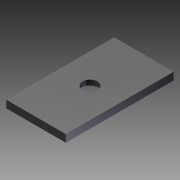
# Autodesk Inventor part: HMEN5-5-dps
Saved by Autodesk Inventor 2015 SP1 (Build 190203100, 203)
## iProperties
Category: Hardware
Company: MISUMI
Created: 2015-02-01
Part Number: HMEN5-5-dps
Catalog Web Link: http://us.misumi-ec.com/vona2/detail/110300479530
Description: HMEN, HMER-door side plate-Latch Magnets for Plate
Vendor: MISUMI
Document SubType Name: Modeling
Designer: psAdmin
Manufacturer: MISUMI
Mass: 0.89831 g
Surface Area: 11.0294 cm^2
Volume: 0.89831 cm^3
Density: 1 g/cm^3
Material: Generic
Appearance: PSOLRGB-192-192-192
Stock Number: HMEN5-5
PSOL_IDENT_0: {\\10.0.0.236\data_v8\23d-libs\misumi\metric\39_accessories_for_al_extrusions\hmen_door_side_plate.p
PSOL_IDENT_1: rj},186 {VTYP=3D},{NB=HMEN5-5-dps},{LINA=HMEN5-5-dps},{NN=HMEN, HMER-door side plate},{DATE=17.11.20
PSOL_IDENT_2: 14 05:31:12},{GEOMDATE=25.05.2009 11:35:00},{VERSION=},{LINEID=10},{LINESUBID=-1},{WBVAR=TS}  {NB=HM
PSOL_IDENT_3: EN5-5-dps},{LINA=HMEN5-5-dps},{KT=DUMMY},{PN=HMEN5-5},{TYPE=HMEN},{TS=HMEN},{NO=5-5}
SUPPLIER: MISUMI
ARTICLENO: HMEN5-5-dps
BOMINFO: HMEN5-5-dps
CREATOR: CADENAS GmbH
Title: HMEN5-5-dps
Author: Misumi
Comments: Latch Magnets for Plate
Autodesk Inventor part; units mm, degrees
sketch "Sketch_1" plane through (0, 0, 0) normal (0, 0, 1) x (1, 0, 0)
  line L0 (-8, 14.5) -> (-8, -14.5)
  line L1 (-8, -14.5) -> (8, -14.5)
  line L2 (8, -14.5) -> (8, 14.5)
  line L3 (8, 14.5) -> (-8, 14.5)
  constraints: 8 end point
extrude "Extrusion1" add sketch "Sketch_1" against normal blind 2
sketch "Sketch_2" plane through (0, 0, 0) normal (1, 0, 0) x (0, 1, 0)
  line L0 (0, -2) -> (0, 0)
  line L1 (0, 0) -> (2, 0)
  line L2 (2, 0) -> (2, -1.2)
  line L3 (2, -1.2) -> (2.8, -2)
  line L4 (2.8, -2) -> (0, -2)
  line L5 (0, -2) -> (0, 0)
  constraints: 12 end point
revolve "Revolution1" cut sketch "Sketch_2" angle 360 about axis through (0, 0, -2) along (0, 0, -1)
ref_plane "to_magnet_XY" through (0, 0, 0) normal (0, 0, 1) x (1, 0, 0)
ref_plane "to_magnet_YZ" through (0, 0, 0) normal (1, 0, 0) x (0, 1, 0)
ref_plane "to_magnet_ZX" through (0, 0, 0) normal (0, 1, 0) x (0, 0, 1)
ref_plane "b1_XY" through (0, -25, -1.2) normal (0, 0, 1) x (1, 0, 0)
ref_plane "b1_YZ" through (0, -25, -1.2) normal (1, 0, 0) x (0, 1, 0)
ref_plane "b1_ZX" through (0, -25, -1.2) normal (0, 1, 0) x (0, 0, 1)
ref_plane "b2_XY" through (0, 25, -1.2) normal (0, 0, 1) x (1, 0, 0)
ref_plane "b2_YZ" through (0, 25, -1.2) normal (1, 0, 0) x (0, 1, 0)
ref_plane "b2_ZX" through (0, 25, -1.2) normal (0, 1, 0) x (0, 0, 1)
ref_plane "bb1_XY" through (0, 0, -1.2) normal (0, 0, 1) x (1, 0, 0)
ref_plane "bb1_YZ" through (0, 0, -1.2) normal (1, 0, 0) x (0, 1, 0)
ref_plane "bb1_ZX" through (0, 0, -1.2) normal (0, 1, 0) x (0, 0, 1)
ref_plane "b2x_XY" through (0, 25, 0) normal (0, 0, 1) x (1, 0, 0)
ref_plane "b2x_YZ" through (0, 25, 0) normal (1, 0, 0) x (0, 1, 0)
ref_plane "b2x_ZX" through (0, 25, 0) normal (0, 1, 0) x (0, 0, 1)
ref_plane "b1x_XY" through (0, -25, 0) normal (0, 0, 1) x (1, 0, 0)
ref_plane "b1x_YZ" through (0, -25, 0) normal (1, 0, 0) x (0, 1, 0)
ref_plane "b1x_ZX" through (0, -25, 0) normal (0, 1, 0) x (0, 0, 1)
body "Solid1"
